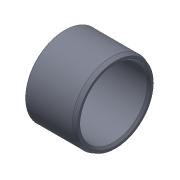
# Autodesk Inventor part: NA-45-h-Crown-157
Saved by Autodesk Inventor 2020.2 (Build 242310000, 310)
## iProperties
Created: 2020-04-21
Part Number: NA-45-h-Crown-157
Material: 19 573.4
Document SubType Name: Modeling
Designer: Jurek
Mass: 61.1006 g
Surface Area: 60.5809 cm^2
Volume: 7.78352 cm^3
Density: 7.85 g/cm^3
Appearance: RAL 7040 Window Grey(2)
Description: Plovoucí chyták
User Status: Ke kontrole
Category: B
Hmotnost (kg): 0,06
Rozmer_A: 38,67
Rozmer_B: 0
Rozmer_C: 0
Rozmer_D: 25
Rada vyrobku: 4100
Prumer nadobky: 45
Cislo artiklu: 4451101303
C. variantniho vykresu: NA-45-h-Crown-157
Jednotka: ks
Cisty rozmer: =Ø<Rozmer_A> - <Rozmer_D>
Predpona: Ø
Stroj na lince: Stahovací lis
RAZ Poznamka 1: ISO 2768-mH
RAZ Poznamka 2: NEOZNAČENÉ HRANY OJEHLIT
RAZ Poznamka 3: KALIT A POPUSTIT NA 58 - 60 HRc
DXF: Ne
QAD_code: M
Rizeni davek: L
Author: Jurek
Revision Number: 00
Autodesk Inventor part; units mm, degrees
ref_plane "YZ Plane" through (0, 0, 0) normal (1, 0, 0) x (0, 1, 0)
ref_plane "XZ Plane" through (0, 0, 0) normal (0, 1, 0) x (-1, 0, 0)
ref_plane "XY Plane" through (0, 0, 0) normal (0, 0, 1) x (1, 0, 0)
sketch "Náčrt1" plane through (0, 0, 0) normal (0, 0, 1) x (1, 0, 0)
  line L0 (0, 0) -> (33.3333, 0)
  line L1 (0, 19.335) -> (25, 19.335)
  line L2 (25, 19.335) -> (25, 16.5)
  line L3 (25, 16.5) -> (0, 16.5)
  line L4 (0, 16.5) -> (0, 19.335)
  dimension "d0" = 25
  dimension "d6" = 38.67
  dimension "d7" = 33
  constraints: 10 end point, 3 perpendicular, 2 horizontal
  measures "d0" distance between parallel lines of L2 L4
  measures "d6" diameter of L1 L0
  measures "d7" diameter of L3 L0
revolve "Rotace1" add sketch "Náčrt1" angle 360 about axis through (0, 0, 0) along (1, 0, 0)
chamfer "Zkosení1" distance 1 angle 45 2 edges at (25, -16.5, 0) (0, -16.5, 0)
chamfer "Zkosení2" distance 0.2 angle 45 1 edges at (0, -19.335, 0)
chamfer "Zkosení4" distance 2 angle 20 1 edges at (25, -19.335, 0) measured on face at (16.7333, 19.2723, -1.5558)
equation "\"Rozmer_A\" = d6"
equation "\"Rozmer_B\" = 0"
equation "\"Rozmer_C\" = 0"
equation "\"Rozmer_D\" = d0"
